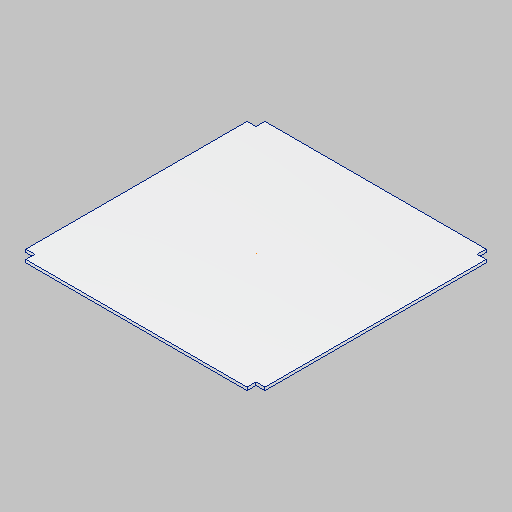
# Autodesk Inventor part: plate1
Saved by Autodesk Inventor 2026.2 (Build 302298000, 298)
## iProperties
Created: 2026-02-25
Part Number: plate1
Material: 알루미늄 6061
Document SubType Name: Modeling
Designer: mjbhang
Density: 2.7 g/cm^3
Appearance: 알루미늄 - 평지
Author: mjbhang
Autodesk Inventor part; units mm, degrees
ref_plane "YZ Plane" through (0, 0, 0) normal (1, 0, 0) x (0, 1, 0)
ref_plane "XZ Plane" through (0, 0, 0) normal (0, 1, 0) x (-1, 0, 0)
ref_plane "XY Plane" through (0, 0, 0) normal (0, 0, 1) x (1, 0, 0)
sketch "스케치1" plane through (0, 0, 0) normal (0, 1, 0) x (-1, 0, 0)
  line L0 (370, -400) -> (-370, -400)
  line L1 (-370, -400) -> (-370, -370)
  line L2 (-370, -370) -> (-400, -370)
  line L3 (-400, -370) -> (-400, 370)
  line L4 (-400, 370) -> (-370, 370)
  line L5 (-370, 370) -> (-370, 400)
  line L6 (-370, 400) -> (370, 400)
  line L7 (370, 400) -> (370, 370)
  line L8 (370, 370) -> (400, 370)
  line L9 (400, 370) -> (400, -370)
  line L10 (400, -370) -> (370, -370)
  line L11 (370, -400) -> (370, -370)
  point P0 (0, 0)
  dimension "d6" = 740
  dimension "d7" = 740
  dimension "d8" = 30
  dimension "d9" = 30
  dimension "d10" = 30
  dimension "d11" = 30
  dimension "d12" = 30
  dimension "d13" = 30
  dimension "d14" = 30
  dimension "d15" = 30
  dimension "d17" = 400
  dimension "d18" = 400
  constraints: 24 end point, 8 perpendicular, 7 point on line, 1 horizontal
  measures "d6" distance of L0.start L0.end
  measures "d7" distance of L8.end L9.end
  measures "d8" distance of L6.end L7.end
  measures "d9" distance of L7.end L8.end
  measures "d10" distance of L3.end L4.end
  measures "d11" distance of L4.end L5.end
  measures "d12" distance of L0.start L10.end
  measures "d13" distance of L9.end L10.end
  measures "d14" distance of L1.end L2.end
  measures "d15" distance of L0.end L1.end
  measures "d17" distance from line of point (0, 0) L3
  measures "d18" distance from line of point (0, 0) L0
extrude "돌출1" add sketch "스케치1" along normal blind 10
